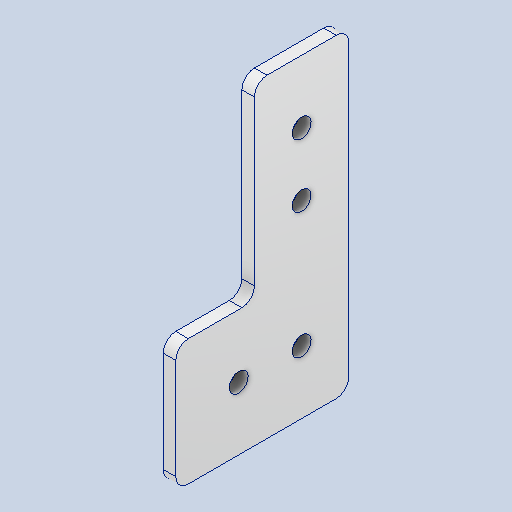
# Autodesk Inventor part: base_weel-v2-Plate-8
Saved by Autodesk Inventor 2025.2 (Build 292293000, 293)
## iProperties
Created: 2025-01-14
Part Number: base_weel-v2-Plate-8
Material: アルミニウム 6061
Document SubType Name: Modeling
Designer: haruy
Density: 2.7 g/cm^3
Appearance: アルミニウム - フラット
Author: haruy
Autodesk Inventor part; units mm, degrees
ref_plane "YZ Plane" through (0, 0, 0) normal (1, 0, 0) x (0, 1, 0)
ref_plane "XZ Plane" through (0, 0, 0) normal (0, 1, 0) x (-1, 0, 0)
ref_plane "XY Plane" through (0, 0, 0) normal (0, 0, 1) x (1, 0, 0)
sketch "スケッチ1" plane through (0, 0, 0) normal (1, 0, 0) x (0, 1, 0)
  line L0 (-114.0211, -198.214) -> (-114.0211, 205.786)
  line L1 (-114.0211, 122.786) -> (139.9789, 122.786)
  line L2 (139.9789, 122.786) -> (139.9789, 107.786)
  line L3 (139.9789, 107.786) -> (-114.0211, 107.786)
  line L4 (-114.0211, 107.786) -> (-114.0211, 122.786)
  line L5 (-74.0211, 147.286) -> (134.9789, 147.286)
  line L6 (134.9789, 147.286) -> (134.9789, -139.714)
  line L7 (134.9789, -139.714) -> (-74.0211, -139.714)
  line L8 (-74.0211, -139.714) -> (-74.0211, 147.286)
  line L9 (-134.0211, -198.214) -> (-134.0211, 205.786)
  line L10 (-134.0211, 3.786) -> (-114.0211, 3.786)
  line L11 (-114.0211, 205.786) -> (-134.0211, 205.786)
  line L12 (-114.0211, -115.214) -> (139.9789, -115.214)
  line L13 (139.9789, -100.214) -> (-114.0211, -100.214)
  line L14 (139.9789, -115.214) -> (139.9789, -100.214)
  line L15 (92.4789, 157.286) -> (82.4789, 157.286)
  line L16 (82.4789, 157.286) -> (82.4789, 3.786)
  line L17 (82.4789, 3.786) -> (92.4789, 3.786)
  line L18 (92.4789, 3.786) -> (92.4789, 157.286)
  line L19 (-21.5211, 157.286) -> (-31.5211, 157.286)
  line L20 (-31.5211, 157.286) -> (-31.5211, 3.786)
  line L21 (-31.5211, 3.786) -> (-21.5211, 3.786)
  line L22 (-21.5211, 3.786) -> (-21.5211, 157.286)
  line L23 (-114.0211, 135.286) -> (-134.0211, 135.286)
  line L24 (-84.0211, 122.786) -> (-84.0211, 107.786)
  circle A0 centre (-124.0211, 115.286) radius 1.5
  circle A1 centre (-124.0211, 125.286) radius 1.5
  line L25 (-114.0211, 135.286) -> (-114.0211, 122.786)
  line L26 (-114.0211, 107.786) -> (-134.0211, 107.786)
  line L27 (-134.0211, 135.286) -> (-134.0211, 107.786)
  circle A2 centre (-104.0211, 115.286) radius 1.5
  circle A3 centre (-94.0211, 115.286) radius 1.5
  line L28 (-84.0211, 107.786) -> (-64.0211, 107.786)
  line L29 (-64.0211, 107.786) -> (-64.0211, 101.786)
  line L30 (-64.0211, 101.786) -> (-84.0211, 101.786)
  line L31 (-84.0211, 101.786) -> (-84.0211, 107.786)
  line L32 (-31.5211, 157.286) -> (-37.5211, 157.286)
  line L33 (-37.5211, 157.286) -> (-37.5211, 137.286)
  line L34 (-37.5211, 137.286) -> (-31.5211, 137.286)
  line L35 (-31.5211, 137.286) -> (-31.5211, 157.286)
  line L36 (92.4789, 157.286) -> (98.4789, 157.286)
  line L37 (98.4789, 157.286) -> (98.4789, 137.286)
  line L38 (98.4789, 137.286) -> (92.4789, 137.286)
  line L39 (92.4789, 137.286) -> (92.4789, 157.286)
  line L40 (30.4789, 147.286) -> (30.4789, -139.714)
  line L41 (134.9789, 3.786) -> (-114.0211, 3.786)
  line L42 (-114.0211, 205.786) -> (-114.0211, -198.214)
  line L43 (-84.0211, -94.214) -> (-84.0211, -100.214)
  line L44 (-64.0211, -94.214) -> (-84.0211, -94.214)
  line L45 (-64.0211, -100.214) -> (-64.0211, -94.214)
  line L46 (-84.0211, -115.214) -> (-84.0211, -100.214)
  circle A4 centre (-94.0211, -107.714) radius 1.5
  circle A5 centre (-104.0211, -107.714) radius 1.5
  circle A6 centre (-124.0211, -107.714) radius 1.5
  circle A7 centre (-124.0211, -117.714) radius 1.5
  line L47 (-114.0211, -127.714) -> (-134.0211, -127.714)
  line L48 (-114.0211, -100.214) -> (-134.0211, -100.214)
  line L49 (-37.5211, -149.714) -> (-37.5211, -129.714)
  line L50 (-31.5211, -149.714) -> (-37.5211, -149.714)
  line L51 (-21.5211, -149.714) -> (-31.5211, -149.714)
  line L52 (-31.5211, -149.714) -> (-31.5211, 3.786)
  line L53 (-21.5211, 3.786) -> (-21.5211, -149.714)
  line L54 (-37.5211, -129.714) -> (-31.5211, -129.714)
  line L55 (82.4789, -149.714) -> (82.4789, 3.786)
  line L56 (92.4789, -149.714) -> (82.4789, -149.714)
  line L57 (92.4789, -149.714) -> (98.4789, -149.714)
  line L58 (98.4789, -149.714) -> (98.4789, -129.714)
  line L59 (98.4789, -129.714) -> (92.4789, -129.714)
  line L60 (92.4789, 3.786) -> (92.4789, -149.714)
  circle A8 centre (-26.5211, 115.286) radius 1.5
  circle A9 centre (87.4789, 115.286) radius 1.5
  circle A10 centre (87.4789, -107.714) radius 1.5
  circle A11 centre (-26.5211, -107.714) radius 1.5
  line L61 (-114.0211, 122.786) -> (-114.0211, 107.786)
  line L62 (-114.0211, -100.214) -> (-114.0211, -115.214)
  point P0 (0, 0)
  point P1 (-114.0211, 3.786)
  point P2 (-114.0211, 3.786)
  point P3 (-114.0211, 107.786)
  dimension "d0" = 15
  dimension "d1" = 287
  dimension "d2" = 209
  dimension "d3" = 83
  dimension "d4" = 10
  dimension "d5" = 10
  dimension "d6" = 30
  dimension "d7" = 3
  dimension "d8" = 7.5
  dimension "d9" = 10
  dimension "d10" = 3
  dimension "d11" = 10
  dimension "d12" = 10
  dimension "d13" = 10
  dimension "d14" = 3
  dimension "d15" = 3
  dimension "d16" = 10
  dimension "d17" = 10
  dimension "d18" = 7.5
  dimension "d19" = 7.5
  dimension "d20" = 6
  dimension "d21" = 10
  dimension "d22" = 10
  dimension "d23" = 5
  dimension "d24" = 143.5
  dimension "d25" = 10
  dimension "d26" = 6
  dimension "d27" = 20
  dimension "d28" = 10
  dimension "d29" = 6
  dimension "d30" = 20
  dimension "d31" = 0
  dimension "d32" = 0
  dimension "d33" = 52
  dimension "d34" = 52
  dimension "d35" = 3
  dimension "d36" = 3
  dimension "d37" = 5
  dimension "d38" = 7.5
  dimension "d39" = 7.5
  dimension "d40" = 5
  constraints: 124 end point, 28 symmetric about line, 14 parallel, 13 perpendicular, 12 centre point, 7 horizontal, 6 point on line, 5 midpoint, 2 collinear, 10 other
  measures "d0" distance of L1.end L2.end
  measures "d1" distance of L5.end L6.end
  measures "d2" distance from line of L8 L41.start
  measures "d3" distance between parallel lines of L11 L1
  measures "d4" distance of L17.end L16.end
  measures "d5" distance of L21.end L20.end
  measures "d6" distance between parallel lines of L24 L0
  measures "d7" diameter of A0
  measures "d8" distance from line of A0.centre L3
  measures "d9" distance from line of A0.centre L9
  measures "d10" diameter of A1
  measures "d11" distance of A0.centre A1.centre
  measures "d12" distance from line of L23 A1.centre
  measures "d13" distance from line of L9 A1.centre
  measures "d14" diameter of A2
  measures "d15" diameter of A3
  measures "d16" distance from line of A2.centre L4
  measures "d17" distance of A3.centre A2.centre
  measures "d18" distance from line of A3.centre L1
  measures "d19" distance from line of A2.centre L1
  measures "d20" distance between parallel lines of L28 L30
  measures "d21" distance between parallel lines of L8 L31
  measures "d22" distance between parallel lines of L8 L29
  measures "d23" distance between parallel lines of L6 L2
  measures "d24" distance between parallel lines of L10 L5
  measures "d25" distance between parallel lines of L5 L19
  measures "d26" distance of L34.end L33.end
  measures "d27" distance of L33.end L32.end
  measures "d28" distance between parallel lines of L15 L5
  measures "d29" distance of L37.end L38.end
  measures "d30" distance of L36.end L37.end
  measures "d31" distance from line of point (-114.021, 3.786) L17
  measures "d32" distance from line of point (-114.021, 3.786) L21
  measures "d33" distance between parallel lines of L22 L40
  measures "d34" distance between parallel lines of L40 L16
  measures "d35" diameter of A8
  measures "d36" diameter of A9
  measures "d37" distance from line of A9.centre L18
  measures "d38" distance from line of A9.centre L1
  measures "d39" distance from line of L1 A8.centre
  measures "d40" distance from line of L22 A8.centre
extrude "押し出し1" add sketch "スケッチ1" against normal blind 2 contours L26 L9 L23 L0 | L0 L1 L24 L3
fillet "フィレット1" radius 2 6 edges at (-1, -84.0211, 122.786) (-1, -84.0211, 107.786) (-1, -114.0211, 122.786) (-1, -114.0211, 135.286) (-1, -134.0211, 135.286) (-1, -134.0211, 107.786)
equation "\"d13\" = d9"
equation "\"d17\" = d16"
equation "\"d19\" = d18"
equation "\"d34\" = d33"
